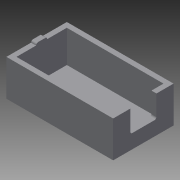
# Autodesk Inventor part: V2_oberteil
Saved by Autodesk Inventor 2015 (Build 190159000, 159)
## iProperties
Created: 2015-05-04
Part Number: V2_oberteil
Material: Generisch
Document SubType Name: Modeling
Designer: krumms
Density: 1 g/cm^3
Appearance: Vorgabe
Author: krumms
Autodesk Inventor part; units mm, degrees
ref_plane "YZ Plane" through (0, 0, 0) normal (1, 0, 0) x (0, 1, 0)
ref_plane "XZ Plane" through (0, 0, 0) normal (0, 1, 0) x (-1, 0, 0)
ref_plane "XY Plane" through (0, 0, 0) normal (0, 0, 1) x (1, 0, 0)
sketch "Skizze1" plane through (0, 0, 0) normal (0, 0, 1) x (1, 0, 0)
  line L0 (0, 0) -> (53, 0)
  line L1 (53, 0) -> (53, 30)
  line L2 (53, 30) -> (0, 30)
  line L3 (0, 30) -> (0, 0)
  dimension "d0" = 30
  dimension "d1" = 53
  constraints: 8 end point, 2 parallel, 1 horizontal, 1 perpendicular
  measures "d0" distance of L2.end L0.start
  measures "d1" distance of L0.start L0.end
extrude "Extrusion1" add sketch "Skizze1" along normal blind 2
sketch "Skizze2" plane through (0, 0, 2) normal (0, 0, 1) x (1, 0, 0)
  line L0 (0, 0) -> (53, 0)
  line L1 (53, 0) -> (53, 30)
  line L2 (53, 30) -> (0, 30)
  line L3 (0, 30) -> (0, 0)
  line L4 (2.5, 2.5) -> (50.5, 2.5)
  line L5 (50.5, 2.5) -> (50.5, 27.5)
  line L6 (50.5, 27.5) -> (2.5, 27.5)
  line L7 (2.5, 27.5) -> (2.5, 2.5)
  dimension "d4" = 25
  dimension "d5" = 48
  dimension "d6" = 2.5
  dimension "d7" = 2.5
  dimension "d8" = 2.5
  dimension "d9" = 2.5
  constraints: 16 end point, 4 parallel, 2 horizontal, 2 perpendicular
  measures "d4" distance of L6.end L4.start
  measures "d5" distance of L4.start L4.end
  measures "d6" distance between parallel lines of L3 L7
  measures "d7" distance between parallel lines of L1 L5
  measures "d8" distance between parallel lines of L0 L4
  measures "d9" distance between parallel lines of L2 L6
extrude "Extrusion2" add sketch "Skizze2" along normal blind 16
sketch "Skizze8" plane through (0, 0, 18) normal (0, 0, 1) x (1, 0, 0)
  line L0 (50.5, 27.5) -> (50.5, 2.5) projected
  line L1 (53, 0) -> (53, 30) projected
  line L2 (50.5, 8.5) -> (53, 8.5)
  line L3 (53, 8.5) -> (53, 21.5)
  line L4 (53, 21.5) -> (50.5, 21.5)
  line L5 (50.5, 21.5) -> (50.5, 8.5)
  line L6 (0, 0) -> (53, 0) projected
  line L7 (53, 30) -> (0, 30) projected
  dimension "d49" = 13
  dimension "d50" = 8.5
  dimension "d51" = 8.5
  constraints: 8 end point, 2 parallel, 2 point on line, 1 horizontal, 1 perpendicular
  measures "d49" distance between parallel lines of L4 L2
  measures "d50" distance between parallel lines of L6 L2
  measures "d51" distance between parallel lines of L7 L4
extrude "Extrusion8" cut sketch "Skizze8" against normal blind 11
hole "Bohrung2" at (17.5, 15, 0) direction (0, 0, 1) diameter 3 end through all countersink diameter 4 countersink angle 90
sketch "Skizze9" plane through (0, 0, 18) normal (0, 0, 1) x (1, 0, 0)
  line L0 (2.5, 27.5) -> (2.5, 2.5) projected
  line L1 (0, 12.25) -> (2.5, 12.25)
  line L2 (2.5, 12.25) -> (2.5, 17.75)
  line L3 (2.5, 17.75) -> (0, 17.75)
  line L4 (0, 17.75) -> (0, 12.25)
  line L5 (0, 0) -> (53, 0) projected
  line L6 (53, 30) -> (0, 30) projected
  dimension "d63" = 5.5
  dimension "d64" = 12.25
  dimension "d65" = 12.25
  constraints: 8 end point, 2 parallel, 1 horizontal, 1 perpendicular, 1 point on line
  measures "d63" distance of L3.end L1.start
  measures "d64" distance between parallel lines of L5 L1
  measures "d65" distance between parallel lines of L6 L3
extrude "Extrusion9" add sketch "Skizze9" along normal blind 1
fillet "Rundung2" radius 1 4 edges at (1.25, 12.25, 19) (1.25, 17.75, 19) (51.75, 21.5, 7) (51.75, 8.5, 7)
